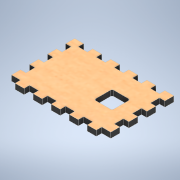
# Autodesk Inventor part: plate_front_small
Saved by Autodesk Inventor 2021 (Build 250183000, 183)
## iProperties
Created: 2021-03-07
Part Number: plate_front_small
Material: Holz (Kirsche)
Document SubType Name: Modeling
Designer: Tilman
Density: 0.63 g/cm^3
Appearance: Glänzend - Schwarz
Author: Tilman
Autodesk Inventor part; units mm, degrees
ref_plane "YZ Plane" through (0, 0, 0) normal (1, 0, 0) x (0, 1, 0)
ref_plane "XZ Plane" through (0, 0, 0) normal (0, 1, 0) x (-1, 0, 0)
ref_plane "XY Plane" through (0, 0, 0) normal (0, 0, 1) x (1, 0, 0)
sketch "Skizze1" plane through (0, 0, 0) normal (0, 1, 0) x (-1, 0, 0)
  line L0 (-5, 0) -> (-5, -3)
  line L1 (-5, -3) -> (0, -3)
  line L2 (-5, 0) -> (-10, 0)
  line L3 (-10, 0) -> (-10, -3)
  line L4 (-10, -3) -> (-15, -3)
  line L5 (-15, 0) -> (-15, -3)
  line L6 (-15, 0) -> (-20, 0)
  line L7 (-20, 0) -> (-20, -3)
  line L8 (-20, -3) -> (-25, -3)
  line L9 (-25, 0) -> (-25, -3)
  line L10 (-25, 0) -> (-30, 0)
  line L11 (-30, 0) -> (-30, -3)
  line L12 (-30, -3) -> (-35, -3)
  line L13 (-35, 0) -> (-35, -3)
  line L14 (-35, 0) -> (-40, 0)
  line L15 (-40, 0) -> (-40, -3)
  line L16 (-40, -3) -> (-45, -3)
  line L17 (-45, 0) -> (-45, -3)
  line L18 (-45, 0) -> (-50, 0)
  line L19 (-50, 0) -> (-50, -3)
  line L20 (-50, -3) -> (-55, -3)
  line L21 (-55, -3) -> (-55, -8)
  line L22 (-55, -8) -> (-52, -8)
  line L23 (-52, -8) -> (-52, -13)
  line L24 (-52, -13) -> (-55, -13)
  line L25 (0, -3) -> (0, -8)
  line L26 (0, -8) -> (-3, -8)
  line L27 (-3, -8) -> (-3, -13)
  line L28 (-3, -13) -> (0, -13)
  line L29 (-52, -18) -> (-52, -23)
  line L30 (-55, -13) -> (-55, -18)
  line L31 (-52, -23) -> (-55, -23)
  line L32 (-55, -18) -> (-52, -18)
  line L33 (-3, -18) -> (-3, -23)
  line L34 (-3, -23) -> (0, -23)
  line L35 (0, -18) -> (-3, -18)
  line L36 (0, -13) -> (0, -18)
  line L37 (0, -38) -> (-5, -38)
  line L38 (-5, -38) -> (-5, -35)
  line L39 (-5, -35) -> (-10, -35)
  line L40 (-10, -35) -> (-10, -38)
  line L41 (-15, -35) -> (-20, -35)
  line L42 (-20, -35) -> (-20, -38)
  line L43 (-10, -38) -> (-15, -38)
  line L44 (-15, -38) -> (-15, -35)
  line L45 (-25, -35) -> (-30, -35)
  line L46 (-30, -35) -> (-30, -38)
  line L47 (-20, -38) -> (-25, -38)
  line L48 (-25, -38) -> (-25, -35)
  line L49 (-35, -35) -> (-40, -35)
  line L50 (-40, -35) -> (-40, -38)
  line L51 (-30, -38) -> (-35, -38)
  line L52 (-35, -38) -> (-35, -35)
  line L53 (-45, -35) -> (-50, -35)
  line L54 (-50, -35) -> (-50, -38)
  line L55 (-40, -38) -> (-45, -38)
  line L56 (-45, -38) -> (-45, -35)
  line L57 (-50, -38) -> (-55, -38)
  line L58 (-35.75, -24) -> (-43.75, -24)
  line L59 (-44.75, -23) -> (-44.75, -15)
  line L60 (-43.75, -14) -> (-35.75, -14)
  line L61 (-34.75, -15) -> (-34.75, -23)
  arc A0 (-35.75, -24) -> (-34.75, -23) centre (-35.75, -23) ccw
  arc A1 (-44.75, -23) -> (-43.75, -24) centre (-43.75, -23) ccw
  arc A2 (-43.75, -14) -> (-44.75, -15) centre (-43.75, -15) ccw
  arc A3 (-34.75, -15) -> (-35.75, -14) centre (-35.75, -15) ccw
  line L62 (-27.5, -38) -> (-27.5, 0) construction
  line L63 (-27.5, -19) -> (-52, -19) construction
  line L64 (-52, -28) -> (-52, -33)
  line L65 (-55, -23) -> (-55, -28)
  line L66 (-52, -33) -> (-55, -33)
  line L67 (-55, -28) -> (-52, -28)
  line L68 (-3, -28) -> (-3, -33)
  line L69 (-3, -33) -> (0, -33)
  line L70 (0, -28) -> (-3, -28)
  line L71 (0, -23) -> (0, -28)
  line L72 (0, -38) -> (0, -33)
  line L73 (-55, -33) -> (-55, -38)
  point P0 (0, 0)
  point P1 (-34.75, -19)
  point P2 (-39.75, -19)
  point P3 (-39.75, -24)
  dimension "d2" = 5
  dimension "d3" = 3
  dimension "d6" = 10
  dimension "d22" = 10
  dimension "d29" = 10
  dimension "d34" = 1
  dimension "d36" = 10
  dimension "d37" = 10
  constraints: 148 end point, 15 equal length, 12 perpendicular, 9 point on line, 8 point on circle, 8 tangent, 8 vertical, 7 horizontal, 5 midpoint, 4 centre point, 3 collinear, 3 equal radius, 3 horizontal alignment, 3 vertical alignment, 1 parallel, 105 other
  measures "d2" distance of L0.start L2.end
  measures "d3" distance of L0.start L0.end
  measures "d6" distance of L0.start L5.start
  measures "d22" distance of L22.end L29.start
  measures "d29" distance of L39.end L41.end
  measures "d34" radius of A0
  measures "d36" distance between parallel lines of L59 L61
  measures "d37" distance between parallel lines of L60 L58
extrude "Extrusion1" add sketch "Skizze1" along normal blind 3
